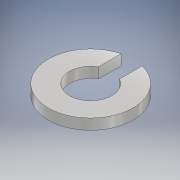
# Autodesk Inventor part: pojistny_krouzek
Saved by Autodesk Inventor 2018 (Build 220112000, 112)
## iProperties
Created: 2023-12-05
Part Number: pojistny_krouzek
Material: Všeobecné
Document SubType Name: Modeling
Designer: 42073
Density: 1 g/cm^3
Appearance: Hliník – leštěný
Author: 42073
Autodesk Inventor part; units mm, degrees
ref_plane "YZ Plane" through (0, 0, 0) normal (1, 0, 0) x (0, 1, 0)
ref_plane "XZ Plane" through (0, 0, 0) normal (0, 1, 0) x (-1, 0, 0)
ref_plane "XY Plane" through (0, 0, 0) normal (0, 0, 1) x (1, 0, 0)
sketch "Náčrt1" plane through (0, 0, 0) normal (0, 0, 1) x (1, 0, 0)
  arc A0 (-0.5, 1.9365) -> (0.5, 1.9365) centre (0, 0) ccw
  arc A1 (-0.5, 0.866) -> (0.5, 0.866) centre (0, 0) ccw
  line L0 (0.5, 0.866) -> (0.5, 1.9365)
  line L1 (-0.5, 1.9365) -> (-0.5, 0.866)
  dimension "d0" = 4
  dimension "d1" = 2
  constraints: 4 end point, 4 point on circle, 2 centre point, 2 coincident
  measures "d0" diameter of A0
  measures "d1" diameter of A1
extrude "Vysunutí1" add sketch "Náčrt1" along normal blind 0.5
